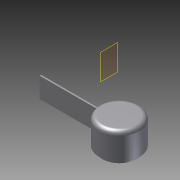
# Autodesk Inventor part: MagBallHolder
Saved by Autodesk Inventor 2012 (Build 160160000, 160)
## iProperties
Created: 2013-07-08
Part Number: MagBallHolder
Material: Default
Document SubType Name: Modeling
Designer: 1
Density: 1 g/cm^3
Author: 1
Autodesk Inventor part; units mm, degrees
ref_plane "XZ Plane" through (0, 0, 0) normal (0, 1, 0) x (-1, 0, 0)
ref_plane "XY Plane" through (0, 0, 0) normal (0, 0, 1) x (1, 0, 0)
sketch "Sketch2" plane through (0, 0, 0) normal (0, 1, 0) x (-1, 0, 0)
  circle A0 centre (0, 0) radius 20
  dimension "d0" = 40
  constraints: 1 centre point, 1 coincident
  measures "d0" diameter of A0
extrude "Extrusion1" add sketch "Sketch2" along normal blind 26.1125
sketch "Sketch3" plane through (0, 0, 0) normal (0, -1, 0) x (1, 0, 0)
  circle A0 centre (0, 0) radius 20 projected
  circle A1 centre (0, 0) radius 17
  dimension "d3" = 3
  constraints: 1 centre point, 1 coincident
  measures "d3" radial gap between concentric circles of A0 A1
extrude "Extrusion2" add sketch "Sketch3" along normal blind 3.3375 contours A1
fillet "Fillet1" radius 4 1 edges at (20, 26.1125, 0)
ref_plane "Work Plane1" through (-20, 0, 0) normal (1, 0, 0) x (0, 1, 0)
sketch "Sketch4" plane through (-20, 0, 0) normal (1, 0, 0) x (0, 1, 0)
  line L0 (21, 0.75) -> (1, 0.75)
  line L1 (1, 0.75) -> (1, -0.75)
  line L2 (1, -0.75) -> (21, -0.75)
  line L3 (21, -0.75) -> (21, 0.75)
  point P0 (0, 0)
  dimension "d7" = 20
  dimension "d8" = 0.75
  dimension "d9" = 0.75
  dimension "d10" = 1
  constraints: 8 end point, 2 parallel, 1 horizontal, 1 perpendicular
  measures "d7" distance between parallel lines of L1 L3
  measures "d8" distance from line of point (0, 0) L0
  measures "d9" distance from line of point (0, 0) L2
  measures "d10" distance from line of point (0, 0) L1
extrude "Extrusion3" add sketch "Sketch4" along normal blind 25.2375 and the other way blind 58.3375
body "Solid1"
